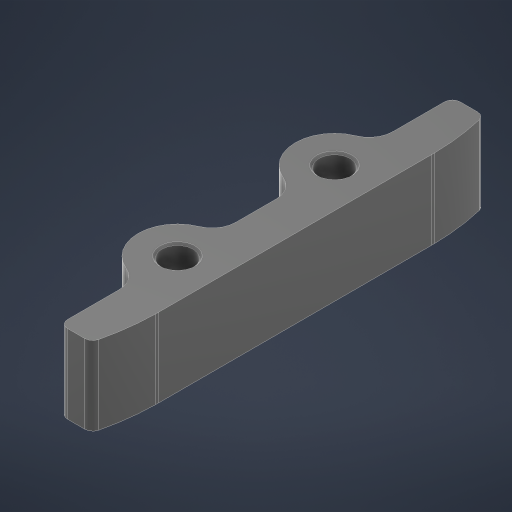
# Autodesk Inventor part: Battery_Slide
Saved by Autodesk Inventor 2025 (Build 290162010, 162A)
## iProperties
Created: 2023-06-20
Part Number: Battery_Slide
Material: Nylon 6/6
Document SubType Name: Modeling
Designer: dzw04
Density: 1.13 g/cm^3
Appearance: Smooth - Black
Author: dzw04
Autodesk Inventor part; units mm, degrees
ref_plane "YZ Plane" through (0, 0, 0) normal (1, 0, 0) x (0, 1, 0)
ref_plane "XZ Plane" through (0, 0, 0) normal (0, 1, 0) x (-1, 0, 0)
ref_plane "XY Plane" through (0, 0, 0) normal (0, 0, 1) x (1, 0, 0)
sketch "Sketch1" plane through (0, 0, 0) normal (0, 1, 0) x (-1, 0, 0)
  circle A0 centre (0, 0) radius 2
  line L0 (0, 0) -> (0, -20) construction
  circle A1 centre (0, -20) radius 2
  arc A2 (0, -5) -> (0, 5) centre (0, 0) ccw
  arc A3 (0, -25) -> (0, -15) centre (0, -20) ccw
  line L1 (0, -5) -> (0, -15)
  line L2 (0, -10) -> (-5, -10) construction
  line L3 (-5, -10) -> (-5, -35) construction
  line L4 (-5, -10) -> (-5, 15) construction
  line L5 (0, 5) -> (0, 15)
  line L6 (0, 15) -> (-4, 15)
  line L7 (0, -25) -> (0, -35)
  line L8 (0, -35) -> (-4, -35)
  line L9 (-5, -10) -> (-5, 7.5)
  line L10 (-5, -10) -> (-5, -27.5)
  arc A4 (-4, 15) -> (-5, 7.5) centre (24.9994, 7.3167) ccw
  arc A5 (-5, -27.5) -> (-4, -35) centre (24.9994, -27.3167) ccw
  dimension "d0" = 4
  dimension "d1" = 20
  dimension "d2" = 4
  dimension "d3" = 10
  dimension "d4" = 10
  dimension "d5" = 5
  dimension "d6" = 25
  dimension "d7" = 25
  dimension "d8" = 10
  dimension "d9" = 4
  dimension "d10" = 10
  dimension "d11" = 4
  dimension "d12" = 17.5
  dimension "d13" = 17.5
  dimension "d14" = 30
  dimension "d15" = 30
  constraints: 22 end point, 8 point on circle, 6 centre point, 5 vertical, 4 coincident, 4 point on line, 2 perpendicular, 1 horizontal, 1 midpoint
  measures "d0" diameter of A0
  measures "d1" distance of L0.start L0.end
  measures "d2" diameter of A1
  measures "d3" diameter of A2
  measures "d4" diameter of A3
  measures "d5" distance of L2.start L2.end
  measures "d6" distance of L2.end L3.end
  measures "d7" distance of L2.end L4.end
  measures "d8" distance of L5.start L5.end
  measures "d9" distance of L5.end L6.end
  measures "d10" distance of L7.start L7.end
  measures "d11" distance of L7.end L8.end
  measures "d12" distance of L2.end L9.end
  measures "d13" distance of L2.end L10.end
  measures "d14" radius of A4
  measures "d15" radius of A5
extrude "Extrusion1" add sketch "Sketch1" along normal blind 10
fillet "Fillet1" radius 3 4 edges at (0, 5, 5) (0, 5, -5) (0, 5, -15) (0, 5, -25)
fillet "Fillet2" radius 1 4 edges at (0, 5, 15) (4, 5, 15) (0, 5, -35) (4, 5, -35)
fillet "Fillet3" radius 25 2 edges at (5, 5, 7.5) (5, 5, -27.5)
chamfer "Chamfer1" distance 0.25 angle 45 4 edges at (2, 10, -20) (2, 10, 0) (2, 0, 0) (2, 0, -20)
body "Solid1"
